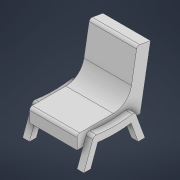
# Autodesk Inventor part: Pieza de practica 14
Saved by Autodesk Inventor 2022 (Build 260153000, 153)
## iProperties
Created: 2022-09-27
Part Number: Pieza de practica 14
Material: Genérico
Document SubType Name: Modeling
Designer: aleon
Density: 1 g/cm^3
Appearance: Valor por defecto
Author: aleon
Autodesk Inventor part; units mm, degrees
ref_plane "YZ Plane" through (0, 0, 0) normal (1, 0, 0) x (0, 1, 0)
ref_plane "XZ Plane" through (0, 0, 0) normal (0, 1, 0) x (-1, 0, 0)
sketch "Boceto1" plane through (0, 0, 0) normal (1, 0, 0) x (0, 1, 0)
  line L0 (85.212, 5.2834) -> (42.3115, 12.8479)
  arc A0 (20, 39.4377) -> (42.3115, 12.8479) centre (47, 39.4377) ccw
  line L1 (20, 39.4377) -> (20, 89)
  line L2 (16, 93) -> (0, 93)
  line L3 (0, 93) -> (0, 0)
  line L4 (0, 0) -> (85.6783, -15.1074)
  line L5 (85.6783, -15.1074) -> (88.4566, 0.6495)
  arc A1 (88.4566, 0.6495) -> (85.212, 5.2834) centre (84.5174, 1.3441) ccw
  arc A2 (20, 89) -> (16, 93) centre (16, 89) ccw
  line L6 (-24, 93) -> (12.0957, 79.8622)
  line L7 (12.0957, 16.1378) -> (-24, 3)
  line L8 (-24, 3) -> (-24, 13)
  line L9 (-24, 13) -> (4.9435, 23.5346)
  line L10 (4.9435, 72.4654) -> (-24, 83)
  line L11 (-24, 83) -> (-24, 93)
  arc A3 (15.327, 74.4007) -> (15.327, 21.5993) centre (186.3007, 48) ccw
  arc A4 (4.9435, 72.4654) -> (4.9435, 23.5346) centre (186.3007, 48) ccw
  arc A5 (15.327, 74.4007) -> (12.0957, 79.8622) centre (10.3856, 75.1638) ccw
  arc A6 (12.0957, 16.1378) -> (15.327, 21.5993) centre (10.3856, 20.8362) ccw
  point P0 (20, 93)
  point P1 (89.1512, 4.5888)
  point P2 (16, 78.4412)
  point P3 (16, 17.5588)
  dimension "d0" = 87
  dimension "d1" = 20
  dimension "d2" = 20
  dimension "d3" = 27
  dimension "d4" = 100
  dimension "d5" = 93
  dimension "d6" = 4
  dimension "d7" = 24
  dimension "d8" = 16
  dimension "d9" = 110
  dimension "d10" = 90
  dimension "d11" = 70
  dimension "d12" = 10
  dimension "d13" = 10
  dimension "d14" = 3
  dimension "d17" = 110
  dimension "d23" = 173
  dimension "d24" = 10
  dimension "d25" = 183
  dimension "d26" = 5
  constraints: 24 end point, 16 point on circle, 10 tangent, 7 centre point, 7 point on line, 4 perpendicular, 2 equal radius, 2 vertical, 2 vertical alignment, 1 coincident, 1 collinear, 1 horizontal alignment, 1 parallel
  measures "d0" distance of L3.end L4.end
  measures "d1" distance of L4.end point (89.151, 4.589)
  measures "d2" distance of point (20, 93) L2.end
  measures "d3" radius of A0
  measures "d4" angle of L4 L3
  measures "d5" distance of L2.end L3.end
  measures "d6" radius of A1
  measures "d7" horizontal distance of L2.end L7.end
  measures "d8" horizontal distance of L2.end point (16, 78.441)
  measures "d9" angle of L11 L10
  measures "d10" distance of L7.end L6.start
  measures "d11" distance of L8.end L10.end
  measures "d12" distance of L10.end L6.start
  measures "d13" distance of L7.end L8.end
  measures "d14" vertical distance of L3.end L7.end
  measures "d17" angle of L8 L9
  measures "d23" radius of A3
  measures "d24" radial gap between concentric circles of A4 A3
  measures "d25" radius of A4
  measures "d26" radius of A5
extrude "Extrusión1" add sketch "Boceto1" against normal blind 70 contours A1 L5 L4 L3 L7 A6 A3 A5 L6 L2 A2 L1 A0 L0 | L3 L9 A4 L10 L6 A5 A3 A6 L7 | L3 L10 A4 L9
extrude "Extrusión2" add sketch "Boceto1" along normal blind 10 contours L7 L8 L9 L3 | L3 L9 A4 L10 L6 A5 A3 A6 L7 | L3 L10 L11 L6
ref_plane "Plano de trabajo1" through (-35, 0, 0) normal (1, 0, 0) x (0, 0, -1)
mirror "Simetría1" about plane through (-35, 0, 0) normal (1, 0, 0) of "Extrusión2"
